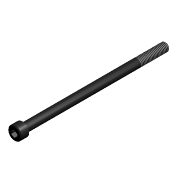
# Autodesk Inventor part: SCREW, SOCKET HD, P, 12.9, M8X1.25X140MM
Saved by Autodesk Inventor 2022.4 (Build 264492000, 492)
## iProperties
Manager: 100-39889
Category: _
Created: 2013-09-04
Material: Steel, Mild
Document SubType Name: Modeling
Designer: cathy.lesperance , Cathy
Density: 7.85 g/cm^3
Checked By: 2FMVY
Engr Approved By: R
User Status: Released
Description: SCREW, SOCKET HD, P, 12.9, M8X1.25X140MM
Mass: 62.4411 g
Surface Area: 41.6133 cm^2
Volume: 7.95428 cm^3
Mfg Approved By: Eric.Michaud
Appearance: Glossy - Black
Part Number: SCREW, SOCKET HD, P, 12.9, M8X1.25X140MM
Control State: 0
Master: False
Checked Out: False
Shininess: 64.0
CN_SERVICEABLE: _
CN_MASS: 0.062441
CL_runCount: 1
FinishProperty: ToBeSet
FIRST_DESCRIPTION: SCREW, SOCKET HD, P, 12.9, M8X1.25X140MM
SECOND_DESCRIPTION: _
THIRD_DESCRIPTION: _
CN_DETAILER: -
CN_MFG_PART_NUM: _
CN_MFG_NAME: DEFAULT
STANDARDCLASSFLAG: R
CUSTOMERNUMBER: _
CN_DESIGNER: Eric.Michaud
PTC_WM_ITERATION: 5
PTC_WM_ORGANIZATION_ID: CLWC
PTC_WM_LIFECYCLE: CLWC_CAD_LC
Density: 0.0
Volumn: 0.0
Area: 0.0
PropertySet Name: Model Information
Author: -
Keywords: DEFAULT
Revision Number: 1
Subject: _
Autodesk Inventor part; units mm, degrees
ref_plane "YZ Plane" through (0, 0, 0) normal (1, 0, 0) x (0, 1, 0)
ref_plane "XZ Plane" through (0, 0, 0) normal (0, 1, 0) x (-1, 0, 0)
ref_plane "XY Plane" through (0, 0, 0) normal (0, 0, 1) x (1, 0, 0)
sketch "Sketch1" plane through (0, 0, 0) normal (0, 0, 1) x (1, 0, 0)
  circle A0 centre (0, 0) radius 4
  dimension "Diameter" = 8
  constraints: 1 centre point
  measures "Diameter" diameter of A0
extrude "Extrusion1" add sketch "Sketch1" along normal blind 140
sketch "Sketch2" plane through (0, 0, 140) normal (0, 0, 1) x (1, 0, 0)
  circle A0 centre (0, 0) radius 4 projected
  circle A1 centre (0, 0) radius 6.5
  dimension "Head_Diameter" = 13
  constraints: 1 centre point, 1 coincident
  measures "Head_Diameter" diameter of A1
extrude "Extrusion2" add sketch "Sketch2" along normal blind 8 contours A0 | A1
sketch "Sketch3" plane through (0, 0, 148) normal (0, 0, 1) x (1, 0, 0)
  circle A0 centre (0, 0) radius 6.5 projected
  circle A1 centre (0, 0) radius 3.4641 construction
  line L0 (0, 3.4641) -> (3, 1.7321)
  line L1 (3, -1.7321) -> (3, 1.7321)
  line L2 (0, 3.4641) -> (-3, 1.7321)
  line L3 (-3, -1.7321) -> (-3, 1.7321)
  line L4 (-3, -1.7321) -> (0, -3.4641)
  line L5 (3, -1.7321) -> (0, -3.4641)
  dimension "Hex_Width" = 6
  constraints: 12 end point, 6 point on circle, 3 equal length, 1 centre point, 1 coincident, 1 parallel, 1 vertical
  measures "Hex_Width" distance between parallel lines of L0 L4
extrude "Extrusion3" cut sketch "Sketch3" against normal blind 4 contours L0 L1 L5 L4 L3 L2
thread "Thread1" size "M8x1.25" class "4g6g" standard "ANSI Metric M Profile" length 28
chamfer "Chamfer1" distance 0.8 angle 45 2 edges at (-6.5, 0, 148) (-4, 0, 0)
equation "\"d9\" = ThreadLength"
equation "\"d12\" = Chamfer"
equation "\"ThreadLength\" = 28"
equation "\"Chamfer\" = 0.8"
body "Solid1"
